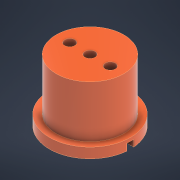
# Autodesk Inventor part: 019
Saved by Autodesk Inventor 2022 (Build 260153000, 153)
## iProperties
Created: 2021-11-15
Part Number: 019
Material: PAEK Plastic
Document SubType Name: Modeling
Designer: vinicius.miguel
Density: 1.32 g/cm^3
Appearance: Smooth - Light Orange
Author: vinicius.miguel
Autodesk Inventor part; units mm, degrees
ref_plane "YZ Plane" through (0, 0, 0) normal (1, 0, 0) x (0, 1, 0)
ref_plane "XZ Plane" through (0, 0, 0) normal (0, 1, 0) x (-1, 0, 0)
ref_plane "XY Plane" through (0, 0, 0) normal (0, 0, 1) x (1, 0, 0)
sketch "Sketch1" plane through (0, 0, 0) normal (0, 0, 1) x (1, 0, 0)
  line L0 (0, 0) -> (0, 18.35)
  line L1 (0, 0) -> (-12, 0)
  line L2 (-12, 0) -> (-12, 3)
  line L3 (-12, 3) -> (-10, 3)
  line L4 (-10, 3) -> (-10, 18.35)
  line L5 (-10, 18.35) -> (0, 18.35)
  dimension "d0" = 20
  dimension "d1" = 24
  dimension "d2" = 3
  dimension "d3" = 18.35
  constraints: 12 end point, 4 perpendicular, 1 horizontal, 1 vertical
  measures "d0" diameter of L4 L0
  measures "d1" diameter of L2 L0
  measures "d2" distance of L1.end L2.end
  measures "d3" distance of L0.start L0.end
revolve "Revolution1" add sketch "Sketch1" angle 360 about axis through (0, 0, 0) along (0, 1, 0)
sketch "Sketch2" plane through (0, 0, 0) normal (0, -1, 0) x (1, 0, 0)
  point P0 (0, 0)
  point P1 (0, 0)
  point P2 (6, 0)
  point P3 (-6, 0)
  dimension "d6" = 6
  dimension "d7" = 6
  constraints: 2 horizontal alignment, 1 coincident
  measures "d6" distance of point (0, 0) point (6, 0)
  measures "d7" distance of point (-6, 0) point (0, 0)
hole "Hole1" at (0, 0, 0) at (6, 0, 0) at (-6, 0, 0) direction (0, 1, 0) diameter 3 end through all counterbore diameter 5 counterbore depth 15
sketch "Sketch3" plane through (0, 0, 0) normal (0, -1, 0) x (1, 0, 0)
  line L0 (-15, 1) -> (15, 1)
  line L1 (15, 1) -> (15, -1)
  line L2 (15, -1) -> (-15, -1)
  line L3 (-15, -1) -> (-15, 1)
  line L4 (-15, 1) -> (15, -1) construction
  line L5 (15, 1) -> (-15, -1) construction
  point P0 (0, 0)
  dimension "d15" = 30
  dimension "d16" = 2
  constraints: 12 end point, 2 midpoint, 2 parallel, 1 horizontal, 1 perpendicular
  measures "d15" distance of L1.end L2.end
  measures "d16" distance of L0.end L1.end
extrude "Extrusion1" cut sketch "Sketch3" against normal blind 2
equation "\"d7\" = d6"
body "Solid1"
